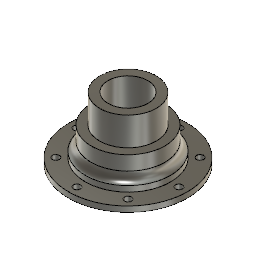
tut1_ coupling flange (Autodesk Fusion 360 design; units mm, degrees)
Autodesk Fusion 360 part; units mm, degrees
sketch "Sketch1" plane through (0, 0, 0) normal (0, 1, 0) x (1, 0, 0)
  line L0 (25.4, -38.1) -> (25.4, -12.7)
  line L1 (25.4, -12.7) -> (33.02, -12.7)
  line L2 (33.02, -12.7) -> (33.02, 0)
  arc A0 (38.1, 7.62) -> (33.02, 0) centre (41.275, 0) ccw
  line L3 (38.1, 7.62) -> (38.1, 12.7)
  line L4 (25.4, -38.1) -> (0, -38.1)
  line L5 (38.1, 12.7) -> (53.34, 12.7)
  line L6 (53.34, 12.7) -> (53.34, 17.78)
  line L7 (53.34, 17.78) -> (0, 17.78)
  line L8 (0, -38.1) -> (0, 17.78)
revolve "Revolve1" add sketch "Sketch1" angle 360 about axis through (0, 0, 38.1) along (0, 0, -1)
sketch "Sketch2" plane through (0, 0, -12.7) normal (0, 0, 1) x (-1, 0, 0)
  circle A0 centre (0, 0) radius 53.34
  circle A1 centre (0, 0) radius 38.1
  circle A2 centre (0, -45.72) radius 3.175
  dimension "d2" = 6.35
  measures "d2" diameter of A2
extrude "Extrude1" cut sketch "Sketch2" against normal up to surface (5.08 mm away) contours A2
pattern_circular "C-Pattern1" count 8 over 360 about axis through (0, 0, 1.75) along (0, 0, 1) of "Extrude1"
sketch "Sketch3" plane through (0, 0, 38.1) normal (0, 0, 1) x (-1, 0, 0)
  circle A0 centre (0, 0) radius 25.4
  circle A1 centre (0, 0) radius 17.78
extrude "Extrude2" cut sketch "Sketch3" against normal up to surface (55.88 mm away) contours A1
